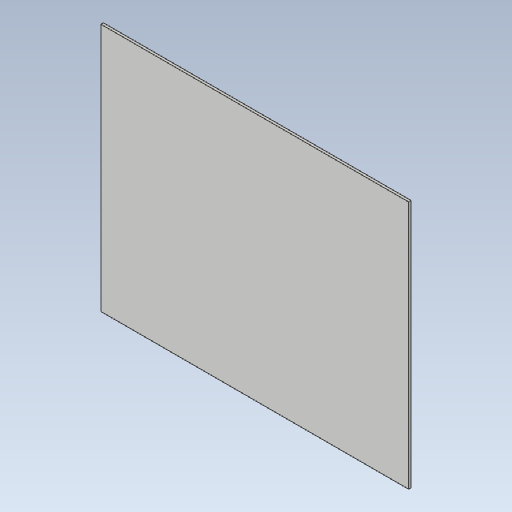
# Autodesk Inventor part: Bottom plate
Saved by Autodesk Inventor 2020 (Build 240168000, 168)
## iProperties
Created: 2019-02-26
Part Number: Bottom plate
Material: Generic
Document SubType Name: Modeling
Designer: LillaHunden
Density: 1 g/cm^3
Appearance: Default
Author: LillaHunden
Autodesk Inventor part; units mm, degrees
ref_plane "YZ Plane" through (0, 0, 0) normal (1, 0, 0) x (0, 1, 0)
ref_plane "XZ Plane" through (0, 0, 0) normal (0, 1, 0) x (-1, 0, 0)
ref_plane "XY Plane" through (0, 0, 0) normal (0, 0, 1) x (1, 0, 0)
sketch "Sketch1" plane through (0, 0, 0) normal (0, 0, 1) x (1, 0, 0)
  line L0 (371, -2) -> (175.4133, -2) construction
  line L1 (371, -2) -> (371, 10) construction
  line L2 (0, 10) -> (371, 10) construction
  line L3 (0, -2) -> (0, 10) construction
  line L4 (0, 10) -> (371, 10)
  line L5 (371, 10) -> (371, -290)
  line L6 (371, -290) -> (0, -290)
  line L7 (0, -290) -> (0, 10)
  line L8 (175.4133, 2) -> (175.4133, -2) projected
  line L9 (108.5867, -2) -> (0, -2) projected
  line L10 (108.5867, -2) -> (108.5867, 2) projected
  line L11 (108.5867, 2) -> (175.4133, 2) projected
  constraints: 8 end point, 2 parallel, 1 horizontal, 1 perpendicular
extrude "Extrusion1" add sketch "Sketch1" along normal blind 3
body "Solid1"
